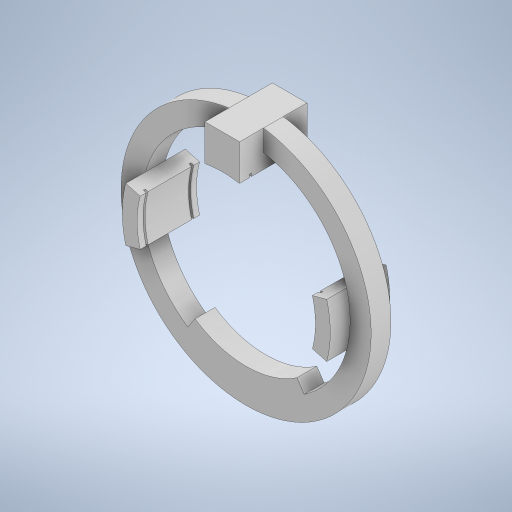
# Autodesk Inventor part: source holder
Saved by Autodesk Inventor 2024 (Build 280153000, 153)
## iProperties
Created: 2025-04-04
Part Number: source holder
Material: Generic
Document SubType Name: Modeling
Designer: NIKHIL
Density: 1 g/cm^3
Appearance: Default
Author: NIKHIL
Autodesk Inventor part; units mm, degrees
sketch "Sketch1" plane through (0, 0, 0) normal (0, 0, 1) x (1, 0, 0)
  line L0 (0, 450) -> (0, 610) construction
  line L1 (-77.5, 610) -> (-77.5, 443.2762)
  line L2 (77.5, 610) -> (77.5, 443.2762)
  arc A0 (77.5, 443.2762) -> (-77.5, 443.2762) centre (0, 0) ccw
  line L3 (-77.5, 610) -> (-77.5, 625)
  line L4 (-77.5, 625) -> (77.5, 625)
  line L5 (77.5, 625) -> (77.5, 610)
  dimension "d7" = 15
  constraints: 12 end point, 2 perpendicular, 2 point on circle, 2 vertical, 1 centre point, 1 coincident, 1 parallel
  measures "d7" distance of L1.start L3.end
extrude "Extrusion1" add sketch "Sketch1" along normal blind 220
sketch "Sketch2" plane through (0, 0, 220) normal (0, 0, 1) x (1, 0, 0)
  arc A0 (77.5, 443.2762) -> (-77.5, 443.2762) centre (0, 0) ccw projected
  line L0 (77.5, 443.2762) -> (77.5, 625) projected
  line L1 (77.5, 458.4962) -> (77.5, 625)
  line L2 (77.5, 625) -> (-77.5, 625)
  line L3 (-77.5, 625) -> (-77.5, 458.4962)
  arc A1 (77.5, 458.4962) -> (-77.5012, 458.496) centre (0, 0) ccw
  dimension "d12" = 465
  constraints: 6 end point, 3 point on circle, 2 perpendicular, 1 centre point, 1 coincident, 1 vertical
  measures "d12" radius of A1
extrude "Extrusion2" add sketch "Sketch2" along normal blind 10
sketch "Sketch3" plane through (0, 0, 230) normal (0, 0, 1) x (1, 0, 0)
  arc A0 (77.5, 443.2762) -> (-77.5, 443.2762) centre (0, 0) ccw projected
  arc A1 (77.5, 443.2762) -> (-77.5, 443.2762) centre (0, 0) ccw
  line L0 (-77.5, 625) -> (-77.5, 443.2762) projected
  line L1 (-77.5, 443.2762) -> (-77.5, 625)
  line L2 (-77.5, 625) -> (77.5, 625)
  line L3 (77.5, 625) -> (77.5, 443.2762)
  constraints: 6 end point, 2 perpendicular, 2 point on circle, 1 centre point, 1 coincident, 1 vertical
extrude "Extrusion3" add sketch "Sketch3" along normal blind 50
ref_plane "Work Plane1" through (0, 0, 110) normal (0, 0, 1) x (1, 0, 0)
mirror "Mirror1" about plane through (0, 0, 110) normal (0, 0, 1) of "Extrusion2", "Extrusion3"
ref_plane "Work Plane2" through (-77.5, 605, 280) normal (0, 1, 0) x (1, 0, 0)
sketch "Sketch4" plane through (-77.5, 605, 280) normal (0, 1, 0) x (1, 0, 0)
  line L0 (5, 15) -> (5, 325)
  line L1 (150, 15) -> (150, 325)
  line L2 (155, 340) -> (155, 0) projected
  line L3 (150, 15) -> (5, 15)
  line L4 (150, 325) -> (5, 325)
  point P0 (77.5, 280)
  constraints: 8 end point, 2 horizontal, 2 vertical
extrude "Extrusion4" cut sketch "Sketch4" against normal up to next
sketch "Sketch5" plane through (77.5, 443.2762, 220) normal (1, 0, 0) x (0, 0, -1)
  line L0 (280, 181.7238) -> (-60, 181.7238) projected
  line L1 (-60, 181.7238) -> (280, 181.7238)
  line L2 (-10, 0) -> (-60, 0) projected
  line L3 (-60, 0) -> (-60, 181.7238)
  line L4 (230, 0) -> (280, 0) projected
  line L5 (280, 181.7238) -> (280, 0) projected
  line L6 (280, 0) -> (280, 181.7238)
  line L7 (230, 0) -> (280, 0)
  line L8 (220, 15.22) -> (230, 15.22) projected
  line L9 (230, 0) -> (230, 15.22)
  line L10 (230, 15.22) -> (220, 15.22)
  line L11 (220, 15.22) -> (220, 0)
  line L12 (0, 16.0372) -> (0, 15.22) projected
  line L13 (0, 0) -> (0, 15.22)
  line L14 (0, 15.22) -> (-10, 15.22) projected
  line L15 (0, 15.22) -> (-10, 15.22)
  line L16 (-10, 15.22) -> (-10, 0)
  line L17 (-60, 0) -> (-10, 0)
  line L18 (0, 0) -> (220, 0)
  point P0 (220, -443.2762)
  constraints: 24 end point, 5 collinear, 4 perpendicular, 3 vertical, 1 point on line
extrude "Extrusion5" add sketch "Sketch5" along normal blind 10
mirror "Mirror2" about plane through (0, 0, 0) normal (1, 0, 0) of "Extrusion5"
ref_plane "Work Plane4" through (0, 0, 110) normal (0, 0, 1) x (1, 0, 0)
sketch "Sketch7" plane through (0, 0, 110) normal (0, 0, 1) x (1, 0, 0)
  line L0 (87.5, 625) -> (87.5, 443.2762) projected
  arc A0 (-87.5, 625) -> (87.5, 625) centre (0, 0) ccw
  arc A1 (-87.5, 517.657) -> (87.5, 517.657) centre (0, 0) ccw
  line L1 (87.5, 517.657) -> (87.5, 625)
  line L2 (-87.5, 625) -> (-87.5, 517.657)
  dimension "d20" = 1050
  constraints: 4 end point, 4 point on circle, 2 centre point, 2 coincident, 1 collinear, 1 parallel, 1 point on line
  measures "d20" diameter of A1
extrude "Extrusion6" add sketch "Sketch7" along normal mid plane 100
sketch "Sketch8" plane through (0, 0, 160) normal (0, 0, 1) x (1, 0, 0)
  line L0 (0, 0) -> (-251.6368, -373.0669) construction
  line L1 (0, 0) -> (0, -450) construction
  line L2 (0, 0) -> (251.6368, -373.0669) construction
  line L3 (0, 0) -> (0, -450) construction
  line L4 (257.2287, -381.3573) -> (293.5763, -435.2447)
  arc A0 (-87.5, 517.657) -> (87.5, 517.657) centre (0, 0) ccw projected
  line L5 (-257.2287, -381.3573) -> (-293.5763, -435.2447)
  arc A1 (-293.5763, -435.2447) -> (293.5763, -435.2447) centre (0, 0) ccw
  arc A2 (0, -460) -> (257.2287, -381.3573) centre (0, 0) ccw
  arc A3 (-257.2287, -381.3573) -> (0, -460) centre (0, 0) ccw
  dimension "d24" = 34
  dimension "d25" = 34
  dimension "d28" = 450
  dimension "d29" = 460
  constraints: 12 end point, 9 point on circle, 5 coincident, 3 centre point, 1 point on line
  measures "d24" angle of L0 L1
  measures "d25" angle of L3 L2
  measures "d28" distance of L0.start L1.end
  measures "d29" radius of A2
extrude "Extrusion7" add sketch "Sketch8" against normal blind 100
sketch "Sketch9" plane through (0, 0, 110) normal (0, 0, 1) x (1, 0, 0)
  arc A0 (293.5763, -435.2447) -> (87.5, 517.657) centre (0, 0) ccw projected
  arc A1 (507.1111, -135.88) -> (507.1111, 135.88) centre (0, 0) ccw
  line L0 (0, 0) -> (507.1111, 135.88) construction
  line L1 (0, 0) -> (525, 0) construction
  line L2 (0, 0) -> (507.1111, -135.88) construction
  arc A2 (434.6666, -116.4686) -> (434.6666, 116.4686) centre (0, 0) ccw
  line L3 (0, 0) -> (434.6666, 116.4686) construction
  line L4 (0, 0) -> (450, 0) construction
  line L5 (0, 0) -> (434.6666, -116.4686) construction
  line L6 (434.6666, 116.4686) -> (507.1111, 135.88)
  line L7 (507.1111, -135.88) -> (434.6666, -116.4686)
  dimension "d30" = 15
  dimension "d31" = 30
  dimension "d32" = 450
  dimension "d33" = 15
  dimension "d34" = 30
  constraints: 16 end point, 6 point on circle, 2 centre point, 2 coincident, 2 equal length, 2 horizontal
  measures "d30" angle of L1 L0
  measures "d31" angle of L2 L0
  measures "d32" radius of A2
  measures "d33" angle of L4 L3
  measures "d34" angle of L5 L3
extrude "Extrusion8" add sketch "Sketch9" along normal mid plane 220
sketch "Sketch10" plane through (0, 0, 220) normal (0, 0, 1) x (1, 0, 0)
  line L0 (507.1111, 135.88) -> (434.6666, 116.4686) projected
  arc A0 (449.1555, -120.3509) -> (449.1555, 120.3509) centre (0, 0) ccw
  arc A1 (507.1111, -135.88) -> (507.1111, 135.88) centre (0, 0) ccw projected
  arc A2 (507.1111, -135.88) -> (507.1111, 135.88) centre (0, 0) ccw
  line L1 (449.1555, 120.3509) -> (507.1111, 135.88)
  line L2 (507.1111, -135.88) -> (449.1555, -120.3509)
  dimension "d37" = 465
  constraints: 4 end point, 4 point on circle, 2 centre point, 2 coincident, 1 collinear, 1 point on line
  measures "d37" radius of A0
extrude "Extrusion9" add sketch "Sketch10" along normal blind 10
sketch "Sketch11" plane through (0, 0, 230) normal (0, 0, 1) x (1, 0, 0)
  arc A0 (434.6666, -116.4686) -> (434.6666, 116.4686) centre (0, 0) ccw projected
  line L0 (434.6666, 116.4686) -> (507.1111, 135.88) projected
  arc A1 (434.6666, -116.4686) -> (434.6666, 116.4686) centre (0, 0) ccw
  arc A2 (507.1111, -135.88) -> (507.1111, 135.88) centre (0, 0) ccw projected
  arc A3 (507.1111, -135.88) -> (507.1111, 135.88) centre (0, 0) ccw
  line L1 (507.1111, 135.88) -> (434.6666, 116.4686)
  line L2 (507.1111, -135.88) -> (434.6666, -116.4686) projected
  line L3 (507.1111, -135.88) -> (434.6666, -116.4686)
  constraints: 4 end point, 4 point on circle, 2 centre point, 2 coincident, 2 collinear
extrude "Extrusion10" add sketch "Sketch11" along normal blind 30
mirror "Mirror3" about plane through (0, 0, 110) normal (0, 0, 1) of "Extrusion9", "Extrusion10"
mirror "Mirror4" about plane through (0, 0, 0) normal (1, 0, 0) of "Extrusion8", "Extrusion9", "Extrusion10", "Mirror3"
ref_plane "Work Plane3" through (0, 0, 0) normal (1, 0, 0) x (0, 1, 0)
body "Solid1"
